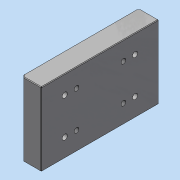
# Autodesk Inventor part: BC-10022
Saved by Autodesk Inventor 2016 (Build 200138000, 138)
## iProperties
Created: 2015-12-01
Part Number: BC-10022
Project: DIPOLO BC-3T- SIRIUS
Cost Center: 1504002005
Material: Aço Carbono AISI 1006
Document SubType Name: Modeling
Designer: reinaldo.basilio
Density: 7.87 g/cm^3
Appearance: Steel
Mass: 813.083 g
Surface Area: 195.053 cm^2
Volume: 103.314 cm^3
Description: Ajustador do gradiente quadrupolar do dipolo BC.
RuleStatus: InUse
AfterMaterialChange0: file://_iMaterial
AfterAnyiPropertyChange0: file://_iMaterial
AfterDocNew0: file://_Naming_par
AfterDocNew1: file://_NameStart
AfterDocNew2: file://_NameStart1
AfterDocNew3: file://_Materiais
DocNumber: XXXXX-XXX-XXXX-00-001.ipt
Folder: .
Title: DIPOLO BC-3T- SIRIUS
Author: reinaldo.basilio
Subject: BC-10022
Autodesk Inventor part; units mm, degrees
ref_plane "YZ Plane" through (0, 0, 0) normal (1, 0, 0) x (0, 1, 0)
ref_plane "XZ Plane" through (0, 0, 0) normal (0, 1, 0) x (-1, 0, 0)
ref_plane "XY Plane" through (0, 0, 0) normal (0, 0, 1) x (1, 0, 0)
sketch "Sketch5" plane through (0, 0, 0) normal (0, 0, 1) x (1, 0, 0)
  line L0 (-50, -8.5) -> (50, -8.5)
  line L1 (50, 8.5) -> (50, -8.5)
  line L2 (-50, 8.5) -> (50, 8.5)
  line L3 (-50, 8.5) -> (-50, -8.5)
  point P0 (0, 0)
  point P1 (0, 8.5)
  point P2 (50, 0)
  dimension "d8" = 100
  dimension "d9" = 17
  constraints: 8 end point, 2 midpoint, 1 horizontal alignment, 1 vertical alignment
  measures "d8" distance of L2.start L1.start
  measures "d9" distance of L1.start L0.end
extrude "Extrusion5" add sketch "Sketch5" along normal mid plane 62.5
chamfer "Chamfer1" distance 2 angle 45 2 edges at (50, -8.5, 0) (-50, -8.5, 0)
sketch "Sketch7" plane through (-48, -8.5, -31.25) normal (0, -1, 0) x (1, 0, 0)
  circle A0 centre (78, 15.75) radius 2.2423
  circle A1 centre (78, 46.75) radius 2.2423
  circle A2 centre (18, 15.75) radius 2.2423
  circle A3 centre (18, 46.75) radius 2.2423
  point P0 (48, 31.25)
  point P1 (96, 0)
  point P2 (96, 62.5)
  dimension "d18" = 60
  dimension "d19" = 30
  dimension "d20" = 31
  dimension "d21" = 15.5
  dimension "d48" = 62.5
  constraints: 4 centre point, 3 equal radius, 2 horizontal alignment, 2 vertical alignment
  measures "d18" distance of A2.centre A0.centre
  measures "d19" horizontal distance of point (48, 31.25) A0.centre
  measures "d20" distance of A1.centre A0.centre
  measures "d21" vertical distance of point (48, 31.25) A0.centre
  measures "d48" distance of point (96, 62.5) point (96, 0)
hole "Hole1" at (30, -8.5, -15.5) at (30, -8.5, 15.5) at (-30, -8.5, 15.5) at (-30, -8.5, -15.5) direction (0, 1, 0) diameter 4.5 end through all counterbore diameter 8 counterbore depth 4.5 clearance for "Socket Head Cap Screw DIN EN ISO 4762" size "M4" standard "DIN"
sketch "Sketch9" plane through (-48, -8.5, -31.25) normal (0, -1, 0) x (1, 0, 0)
  circle A0 centre (78, 15.75) radius 4 projected
  circle A1 centre (78, 46.75) radius 4 projected
  circle A2 centre (68, 46.75) radius 2.5
  circle A3 centre (68, 15.75) radius 2.5
  line L0 (48, 31.25) -> (48, 8.9232)
  circle A4 centre (28, 46.75) radius 2.5
  circle A5 centre (28, 15.75) radius 2.5
  dimension "d39" = 20
  dimension "d40" = 5
  constraints: 4 centre point, 2 end point, 2 horizontal alignment, 2 symmetric about line, 1 equal radius, 1 vertical, 1 vertical alignment, 2 other
  measures "d39" horizontal distance of A2.centre L0.start
  measures "d40" diameter of A3
hole "Hole3" at (-20, -8.5, -15.5) at (-20, -8.5, 15.5) at (20, -8.5, 15.5) at (20, -8.5, -15.5) direction (0, 1, 0) diameter 4.134 end through all thread size "M5x0.8" class "6H" standard "ISO Metric profile"
chamfer "Chamfer4" distance 0.5 angle 45 14 edges at (0, 8.5, 31.25) (50, 8.5, 0) (-50, 8.5, 0) (0, 8.5, -31.25) (50, 1, 31.25) (50, 1, -31.25) (-50, 1, -31.25) (-50, 1, 31.25) (0, -8.5, 31.25) (0, -8.5, -31.25) (49, -7.5, 31.25) (-49, -7.5, 31.25) (49, -7.5, -31.25) (-49, -7.5, -31.25)
equation "\"d19\" = 0.5 * d18"
equation "\"d21\" = 0.5 * d20"
body "Solid5"
